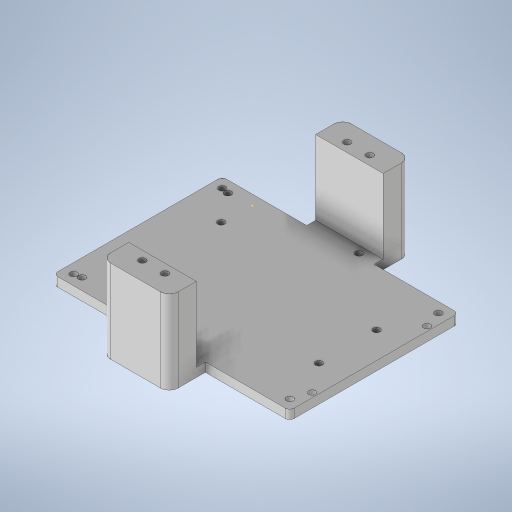
# Autodesk Inventor part: pablo opencr
Saved by Autodesk Inventor 2023 (Build 270158000, 158)
## iProperties
Created: 2022-09-07
Part Number: pablo opencr
Material: Genérico
Document SubType Name: Modeling
Designer: Lab. de Manufactura
Density: 1 g/cm^3
Appearance: Valor por defecto
Author: Lab. de Manufactura
Autodesk Inventor part; units mm, degrees
ref_plane "YZ Plane" through (0, 0, 0) normal (1, 0, 0) x (0, 1, 0)
ref_plane "XZ Plane" through (0, 0, 0) normal (0, 1, 0) x (-1, 0, 0)
ref_plane "XY Plane" through (0, 0, 0) normal (0, 0, 1) x (1, 0, 0)
sketch "Boceto1" plane through (0, 0, 0) normal (0, 1, 0) x (-1, 0, 0)
  line L0 (0, 0) -> (0, -87) construction
  line L1 (0, 0) -> (0, 83.8978) construction
  line L2 (0, 0) -> (-87, 0) construction
  line L3 (0, 0) -> (59, 0) construction
  line L4 (-74.5, -10) -> (-49.5, -10)
  line L5 (-49.5, -10) -> (-49.5, 10)
  line L6 (-49.5, 10) -> (-74.5, 10)
  line L7 (-74.5, 10) -> (-74.5, -10)
  line L8 (-74.5, -10) -> (-49.5, 10) construction
  line L9 (-49.5, -10) -> (-74.5, 10) construction
  line L10 (-18, 63.0769) -> (-64.0145, 27.7688)
  line L11 (9, 69.9829) -> (55.0145, 34.6747)
  line L12 (9, 69.9829) -> (20.2282, 84.6157)
  line L13 (-18, 63.0769) -> (-31.752, 80.9988)
  line L14 (-64.0145, 27.7688) -> (-75.6609, 42.9467)
  line L15 (-18, -63.0769) -> (-64.0145, -27.7688)
  line L16 (9, -69.9829) -> (55.0145, -34.6747)
  line L17 (9, -69.9829) -> (20.2282, -84.6157)
  line L18 (-18, -63.0769) -> (-31.752, -80.9988)
  line L19 (-64.0145, -27.7688) -> (-75.6609, -42.9467)
  arc A0 (-75.6609, 42.9467) -> (-75.6609, -42.9467) centre (0, 0) ccw
  arc A1 (20.2282, 84.6157) -> (-31.752, 80.9988) centre (0, 0) ccw
  arc A2 (-31.752, -80.9988) -> (20.2282, -84.6157) centre (0, 0) ccw
  line L20 (59, 37.9189) -> (59, -37.9189)
  line L21 (58.0583, 38.6415) -> (59, 37.9189)
  line L22 (55.0145, 34.6747) -> (58.0583, 38.6415)
  line L23 (58.0583, -38.6415) -> (59, -37.9189)
  line L24 (55.0145, -34.6747) -> (58.0583, -38.6415)
  circle A3 centre (-18.868, 51.0667) radius 1.5
  circle A4 centre (-52.1888, 25.4987) radius 1.5
  line L25 (-41.0072, 45.4229) -> (-35.5284, 38.2827) construction
  line L26 (-18.868, 51.0667) -> (-52.1888, 25.4987) construction
  line L27 (32.0072, 52.3288) -> (22.9685, 40.5493) construction
  circle A5 centre (9.868, 57.9726) radius 1.5
  circle A6 centre (43.1888, 32.4046) radius 1.5
  circle A7 centre (-18.868, -51.0667) radius 1.5
  circle A8 centre (-52.1888, -25.4987) radius 1.5
  circle A9 centre (9.868, -57.9726) radius 1.5
  circle A10 centre (43.1888, -32.4046) radius 1.5
  line L28 (43.1888, 32.4046) -> (9.868, 57.9726) construction
  point P0 (-62, 0)
  point P1 (-74.5, 0)
  point P2 (26.5284, 45.1886)
  dimension "d1" = 25
  dimension "d2" = 20
  dimension "d9" = 52.5
  dimension "d10" = 52.5
  dimension "d11" = 61
  dimension "d12" = 61
  dimension "d13" = 58
  dimension "d17" = 90
  dimension "d18" = 9
  dimension "d19" = 18
  dimension "d20" = 58
  dimension "d21" = 90
  dimension "d22" = 90
  dimension "d23" = 87
  dimension "d24" = 87
  dimension "d26" = 59
  dimension "d27" = 5
  dimension "d28" = 5
  dimension "d29" = 3
  dimension "d30" = 3
  dimension "d31" = 42
  dimension "d32" = 9
  dimension "d37" = 90
  dimension "d38" = 3
  dimension "d39" = 3
  dimension "d40" = 42
  dimension "d41" = 9
  dimension "d54" = 62
  constraints: 58 end point, 11 centre point, 11 symmetric about line, 9 parallel, 8 point on circle, 7 midpoint, 3 horizontal, 3 vertical, 2 perpendicular, 2 point on line, 1 coincident, 4 other
  measures "d1" distance of L5.end L6.end
  measures "d2" distance of L4.end L5.end
  measures "d9" angle of L1 L11
  measures "d10" angle of L1 L10
  measures "d11" distance from line of point (0, 0) L11
  measures "d12" distance from line of point (0, 0) L10
  measures "d13" distance of L11.start L11.end
  measures "d17" angle of L11 L12
  measures "d18" distance from line of L1 L11.start
  measures "d19" distance from line of L1 L10.start
  measures "d20" distance of L10.start L10.end
  measures "d21" angle of L10 L13
  measures "d22" angle of L10 L14
  measures "d23" radius of A0
  measures "d24" radius of A1
  measures "d26" distance between parallel lines of L0 L20
  measures "d27" distance between parallel lines of L11 L21
  measures "d28" distance between parallel lines of L23 L16
  measures "d29" diameter of A3
  measures "d30" diameter of A4
  measures "d31" distance of L26.end L26.start
  measures "d32" distance from line of L10 L26.start
  measures "d37" angle of L11 L27
  measures "d38" diameter of A5
  measures "d39" diameter of A6
  measures "d40" distance of L28.end L28.start
  measures "d41" distance from line of L11 L28.end
  measures "d54" distance of point (0, 0) point (-62, 0)
extrude "Extrusión1" add sketch "Boceto1" along normal blind 3
sketch "Boceto2" plane through (0, 3, 0) normal (0, 1, 0) x (1, 0, 0)
  line L0 (-55.0145, -34.6747) -> (-9, -69.9829) projected
  line L1 (-32.0072, -52.3288) -> (-0.1642, -10.8301) construction
  circle A0 centre (-33.4486, -19.711) radius 1.55
  circle A1 centre (-0.1278, -45.2789) radius 1.55
  line L2 (-33.4486, -19.711) -> (-0.1278, -45.2789) construction
  circle A2 centre (-43.1888, -32.4046) radius 1.5 construction
  line L3 (18, -63.0769) -> (64.0145, -27.7688) projected
  line L4 (41.0072, -45.4229) -> (14.3892, -10.7335) construction
  circle A3 centre (9.1278, -38.373) radius 1.55
  circle A4 centre (42.4486, -12.805) radius 1.55
  line L5 (42.4486, -12.805) -> (9.1278, -38.373) construction
  circle A5 centre (18.868, -51.0667) radius 1.5 construction
  line L6 (-59, 37.9189) -> (-59, -37.9189) construction
  line L7 (-59, 0) -> (115.874, 0) construction
  circle A6 centre (-33.4486, 19.711) radius 1.55
  circle A7 centre (-0.1278, 45.2789) radius 1.55
  circle A8 centre (9.1278, 38.373) radius 1.55
  circle A9 centre (42.4486, 12.805) radius 1.55
  point P0 (0, 0)
  dimension "d44" = 3.1
  dimension "d45" = 3.1
  dimension "d46" = 21
  dimension "d47" = 42
  dimension "d48" = 16
  dimension "d51" = 16
  dimension "d52" = 21
  dimension "d53" = 42
  constraints: 10 end point, 8 centre point, 4 symmetric about line, 3 midpoint, 2 equal radius, 2 parallel, 2 perpendicular, 1 horizontal, 4 other
  measures "d44" diameter of A0
  measures "d45" diameter of A1
  measures "d46" distance from line of L1 L2.start
  measures "d47" distance of L2.start L2.end
  measures "d48" distance of A2.centre L2.start
  measures "d51" distance from line of L5 A5.centre
  measures "d52" distance from line of L4 L5.end
  measures "d53" distance of L5.start L5.end
extrude "Extrusión2" cut sketch "Boceto2" against normal blind 10
sketch "Boceto3" plane through (0, 3, 0) normal (0, 1, 0) x (1, 0, 0)
  circle A0 centre (0, 0) radius 90 construction
  dimension "d55" = 180
  constraints: 1 centre point, 1 coincident
  measures "d55" diameter of A0
sketch "Boceto5" plane through (0, 3, 0) normal (0, 1, 0) x (1, 0, 0)
  arc A0 (75.6609, -42.9467) -> (75.6609, 42.9467) centre (0, 0) ccw construction
  line L0 (87, 0) -> (-107.1861, 0) construction
  line L1 (-55.0145, -34.6747) -> (-9, -69.9829) projected
  line L2 (-9, -69.9829) -> (5.2804, -80.9406)
  line L3 (5.2804, -80.9406) -> (0.6326, -86.9977)
  arc A1 (-20.2282, -84.6157) -> (31.752, -80.9988) centre (0, 0) ccw projected
  line L4 (31.752, -80.9988) -> (18, -63.0769) projected
  line L5 (18, -63.0769) -> (4.513, -73.4259)
  line L6 (4.513, -73.4259) -> (9.3831, -79.7727)
  line L7 (9.3831, -79.7727) -> (22.8701, -69.4238)
  line L8 (-55.0145, -34.6747) -> (-59, -31.6165)
  line L9 (-59, 37.9189) -> (-59, -37.9189) projected
  circle A2 centre (42.4486, 12.805) radius 1.55 projected
  circle A3 centre (-33.4486, -19.711) radius 1.55 projected
  circle A4 centre (-33.4486, 19.711) radius 1.55 projected
  circle A5 centre (42.4486, -12.805) radius 1.55 projected
  circle A6 centre (9.1278, 38.373) radius 1.55 projected
  circle A7 centre (-0.1278, -45.2789) radius 1.55 projected
  circle A8 centre (-0.1278, 45.2789) radius 1.55 projected
  circle A9 centre (9.1278, -38.373) radius 1.55 projected
  arc A10 (-20.2282, -84.6157) -> (31.752, -80.9988) centre (0, 0) ccw projected
  line L10 (31.752, -80.9988) -> (18, -63.0769) projected
  line L11 (18, -63.0769) -> (64.0145, -27.7688) projected
  line L12 (64.0145, -27.7688) -> (75.6609, -42.9467) projected
  arc A11 (75.6609, -42.9467) -> (75.6609, 42.9467) centre (0, 0) ccw projected
  line L13 (75.6609, 42.9467) -> (64.0145, 27.7688) projected
  line L14 (64.0145, 27.7688) -> (18, 63.0769) projected
  line L15 (18, 63.0769) -> (31.752, 80.9988) projected
  arc A12 (31.752, 80.9988) -> (-20.2282, 84.6157) centre (0, 0) ccw projected
  line L16 (-20.2282, 84.6157) -> (-9, 69.9829) projected
  line L17 (-9, 69.9829) -> (-55.0145, 34.6747) projected
  line L18 (-55.0145, 34.6747) -> (-58.0583, 38.6415) projected
  line L19 (-58.0583, 38.6415) -> (-59, 37.9189) projected
  line L20 (-59, 37.9189) -> (-59, -37.9189) projected
  line L21 (-59, -37.9189) -> (-58.0583, -38.6415) projected
  line L22 (-58.0583, -38.6415) -> (-55.0145, -34.6747) projected
  line L23 (-55.0145, -34.6747) -> (-9, -69.9829) projected
  line L24 (-9, -69.9829) -> (-20.2282, -84.6157) projected
  circle A13 centre (-43.1888, 32.4046) radius 1.5 projected
  circle A14 centre (-9.868, 57.9726) radius 1.5 projected
  circle A15 centre (18.868, 51.0667) radius 1.5 projected
  circle A16 centre (52.1888, 25.4987) radius 1.5 projected
  circle A17 centre (-43.1888, -32.4046) radius 1.5 projected
  circle A18 centre (-9.868, -57.9726) radius 1.5 projected
  circle A19 centre (52.1888, -25.4987) radius 1.5 projected
  circle A20 centre (18.868, -51.0667) radius 1.5 projected
  line L25 (74.5, 10) -> (74.5, -10) projected
  line L26 (74.5, -10) -> (49.5, -10) projected
  line L27 (49.5, -10) -> (49.5, 10) projected
  line L28 (49.5, 10) -> (74.5, 10) projected
  line L29 (18, -63.0769) -> (64.0145, -27.7688) projected
  line L30 (64.0145, -27.7688) -> (78.2949, -16.8111)
  line L31 (78.2949, -16.8111) -> (83.6749, -23.8225)
  point P0 (-9, -69.9829)
  point P1 (-20.2282, -84.6157)
  dimension "d66" = 18
  dimension "d67" = 17
  dimension "d68" = 8
  dimension "d69" = 18
  constraints: 18 end point, 5 perpendicular, 3 collinear, 3 point on circle, 2 point on line, 1 horizontal
  measures "d66" distance of L1.end L2.end
  measures "d67" distance of L4.end L5.end
  measures "d68" distance of L5.end L6.end
  measures "d69" distance of L11.end L30.end
extrude "Extrusión3" cut sketch "Boceto5" against normal blind 10 contours L22 L21 L9 L8 | L2 L3 A1 L24 | L7 L6 L5 L4 | L30 L31 A11 L12
mirror "Simetría1" about plane through (0, 0, 0) normal (0, 0, 1) of "Extrusión3"
sketch "Boceto6" plane through (0, 3, 0) normal (0, 1, 0) x (1, 0, 0)
  line L0 (-59, 31.6165) -> (-59, -31.6165) projected
  line L1 (-59, 0) -> (-50.8, 0)
  line L2 (-50.8, 0) -> (-50.8, 35.5)
  line L3 (-48.8, 37.5) -> (52.2, 37.5)
  line L4 (54.2, 35.5) -> (54.2, -35.5)
  line L5 (-50.8, 0) -> (-50.8, -35.5)
  line L6 (-48.8, -37.5) -> (52.2, -37.5)
  arc A0 (-50.8, -35.5) -> (-48.8, -37.5) centre (-48.8, -35.5) ccw
  arc A1 (-48.8, 37.5) -> (-50.8, 35.5) centre (-48.8, 35.5) ccw
  arc A2 (54.2, 35.5) -> (52.2, 37.5) centre (52.2, 35.5) ccw
  arc A3 (52.2, -37.5) -> (54.2, -35.5) centre (52.2, -35.5) ccw
  point P0 (0, 0)
  point P1 (-50.8, 37.5)
  point P2 (54.2, 37.5)
  point P3 (54.2, -37.5)
  point P4 (-50.8, -37.5)
  dimension "d72" = 8.2
  dimension "d73" = 37.5
  dimension "d74" = 105
  dimension "d75" = 75
  dimension "d76" = 37.5
  dimension "d77" = 105
  dimension "d78" = 2
  constraints: 12 end point, 8 point on circle, 8 point on line, 8 tangent, 4 centre point, 3 equal radius, 2 horizontal, 2 vertical, 1 midpoint, 1 perpendicular
  measures "d72" distance of L1.start L1.end
  measures "d73" distance of L1.end point (-50.8, 37.5)
  measures "d74" distance of point (-50.8, 37.5) point (54.2, 37.5)
  measures "d75" distance of point (54.2, 37.5) point (54.2, -37.5)
  measures "d76" distance of L1.end point (-50.8, -37.5)
  measures "d77" distance of point (-50.8, -37.5) point (54.2, -37.5)
  measures "d78" radius of A0
extrude "Extrusión4" add sketch "Boceto6" along normal blind 4
sketch "Boceto7" plane through (0, 0, 0) normal (0, -1, 0) x (1, 0, 0)
  circle A0 centre (-33.4486, -19.711) radius 1.55 projected
  circle A1 centre (-33.4486, -19.711) radius 1.55
  circle A2 centre (-43.1888, -32.4046) radius 1.5 projected
  circle A3 centre (-43.1888, -32.4046) radius 1.5
  circle A4 centre (-33.4486, 19.711) radius 1.55 projected
  circle A5 centre (-33.4486, 19.711) radius 1.55
  circle A6 centre (-43.1888, 32.4046) radius 1.5 projected
  circle A7 centre (-43.1888, 32.4046) radius 1.5
  circle A8 centre (9.1278, 38.373) radius 1.55 projected
  circle A9 centre (9.1278, 38.373) radius 1.55
  circle A10 centre (9.1278, -38.373) radius 1.55 projected
  circle A11 centre (9.1278, -38.373) radius 1.55
  circle A12 centre (42.4486, -12.805) radius 1.55 projected
  circle A13 centre (42.4486, -12.805) radius 1.55
  circle A14 centre (42.4486, 12.805) radius 1.55 projected
  circle A15 centre (42.4486, 12.805) radius 1.55
  circle A16 centre (52.1888, -25.4987) radius 1.5 projected
  circle A17 centre (52.1888, -25.4987) radius 1.5
  circle A18 centre (52.1888, 25.5678) radius 1.5016
  point P0 (0, 0)
  dimension "d81" = 3.0032
  dimension "d82" = 3
  dimension "d83" = 3.1
  dimension "d84" = 3.1
  dimension "d85" = 3.1
  dimension "d86" = 3.1
  dimension "d87" = 3.1
  dimension "d88" = 3.1
  dimension "d89" = 3
  dimension "d90" = 3
  dimension "d91" = 51.0664
  dimension "d92" = 16.0549
  constraints: 10 centre point, 9 coincident
  measures "d81" diameter of A18
  measures "d82" diameter of A17
  measures "d83" diameter of A15
  measures "d84" diameter of A13
  measures "d85" diameter of A9
  measures "d86" diameter of A11
  measures "d87" diameter of A5
  measures "d88" diameter of A1
  measures "d89" diameter of A7
  measures "d90" diameter of A3
  measures "d91" distance of A16.centre A18.centre
  measures "d92" distance of A14.centre A18.centre
hole "Agujero1" at (-43.1888, 0, -32.4046) at (-33.4486, 0, -19.711) at (-33.4486, 0, 19.711) at (-43.1888, 0, 32.4046) at (9.1278, 0, -38.373) at (42.4486, 0, -12.805) at (42.4486, 0, 12.805) at (52.1888, 0, 25.5678) at (9.1278, 0, 38.373) direction (0, 1, 0) diameter 3 end through all
sketch "Boceto8" plane through (0, 0, 0) normal (0, -1, 0) x (1, 0, 0)
  circle A0 centre (52.1888, -25.4987) radius 1.5 projected
  circle A1 centre (52.1888, -25.4987) radius 1.5
  point P0 (0, 0)
  constraints: 1 centre point, 1 coincident
hole "Agujero2" at (52.1888, 0, -25.4987) direction (0, 1, 0) diameter 3 end through all
sketch "Boceto9" plane through (0, 7, 0) normal (0, 1, 0) x (1, 0, 0)
  circle A0 centre (-46.3, -33.001) radius 2
  line L0 (0, 0) -> (-50.8, 0)
  line L1 (-50.8, 35.5) -> (-50.8, -35.5) projected
  line L2 (0, 0) -> (54.2, 0)
  line L3 (54.2, -10) -> (54.2, 10) projected
  line L4 (0, 0) -> (0, -37.5107)
  line L5 (-50.8, 0) -> (-50.8, -35.5)
  line L6 (-48.8, -37.5) -> (7.908, -37.5) projected
  circle A1 centre (-46.3, 33.001) radius 2
  line L7 (54.2, -10) -> (54.2, -35.2997) projected
  circle A2 centre (49.7, -33) radius 2
  circle A3 centre (49.7, 33) radius 2
  dimension "d109" = 4
  dimension "d114" = 4
  dimension "d118" = 4.5
  dimension "d119" = 70.5
  dimension "d120" = 0.0107
  dimension "d121" = 100.5
  dimension "d122" = 70.501
  constraints: 8 end point, 4 centre point, 2 midpoint, 2 symmetric about line, 2 vertical, 2 other
  measures "d109" diameter of A0
  measures "d114" diameter of A2
  measures "d118" distance from line of A3.centre L3
  measures "d119" distance from line of A3.centre L6
  measures "d120" distance from line of L4.end L6
  measures "d121" distance from line of A1.centre L3
  measures "d122" distance from line of A1.centre L6
hole "Agujero3" at (-46.3, 7, -33.001) at (-46.3, 7, 33.001) at (49.7, 7, -33) at (49.7, 7, 33) direction (0, -1, 0) diameter 3 end through all
sketch "Boceto10" plane through (-59, 0, -31.6165) normal (-1, 0, 0) x (0, 0, 1)
  line L0 (-49.3823, 0) -> (-55.3812, 0) projected
  line L1 (118.6142, 3) -> (118.6142, 0) projected
  line L2 (-55.3812, 0) -> (118.6142, 0)
  line L3 (118.6142, 0) -> (118.6142, 3)
  line L4 (118.6142, 3) -> (-55.3812, 3)
  line L5 (-55.3812, 3) -> (-55.3812, 0)
  point P0 (31.6165, 0)
  point P1 (-49.3823, 0)
  constraints: 8 end point, 2 parallel, 1 horizontal, 1 perpendicular
extrude "Extrusión5" cut sketch "Boceto10" against normal blind 1000
sketch "Boceto11" plane through (-48.8, 3, 37.5) normal (0, 0, 1) x (1, 0, 0)
  line L0 (-2, 0) -> (0, 0) projected
  line L1 (-2, 0) -> (50.5, 0)
  line L2 (56.708, 0) -> (0, 0) construction
  line L3 (50.5, 0) -> (65.5, 0)
  line L4 (50.5, 0) -> (35.5, 0) construction
  line L5 (103, 4) -> (101, 4) projected
  line L6 (103, 4) -> (-2, 4) construction
  line L7 (65.5, 0) -> (65.5, 4)
  line L8 (35.5, 0) -> (35.5, 4)
  line L9 (56.708, 4) -> (0, 4) projected
  line L10 (35.5, 0) -> (50.5, 0)
  line L11 (35.5, 4) -> (65.5, 4)
  line L12 (101, 4) -> (59.1476, 4) projected
  point P0 (48.8, -3)
  point P1 (35.5, 0)
  dimension "d132" = 52.5
  dimension "d133" = 15
  dimension "d134" = 15
  constraints: 16 end point, 4 point on line, 3 horizontal, 2 perpendicular, 1 collinear
  measures "d132" distance of L0.start L1.end
  measures "d133" distance of L1.end L3.end
  measures "d134" distance of L1.end L4.end
extrude "Extrusión6" add sketch "Boceto11" along normal blind 16
sketch "Boceto12" plane through (0, 7, 0) normal (0, 1, 0) x (1, 0, 0)
  line L0 (-50.8, -35.5) -> (-50.8, 35.5) projected
  line L1 (-50.8, 0) -> (54.2, 0)
  line L2 (54.2, -35.5) -> (54.2, 35.5) projected
  line L3 (-13.3, -37.5) -> (-13.3, -53.5) projected
  line L4 (-13.3, -37.5) -> (-13.3, -53.5)
  line L5 (-13.3, -53.5) -> (16.7, -53.5) projected
  line L6 (-13.3, -53.5) -> (16.7, -53.5)
  line L7 (16.7, -53.5) -> (16.7, -37.5)
  line L8 (16.7, -37.5) -> (-13.3, -37.5)
  line L9 (-13.3, 37.5) -> (-13.3, 53.5)
  line L10 (-13.3, 53.5) -> (16.7, 53.5)
  line L11 (16.7, 53.5) -> (16.7, 37.5)
  line L12 (16.7, 37.5) -> (-13.3, 37.5)
  point P0 (0, 0)
  constraints: 18 end point, 4 symmetric about line, 3 perpendicular, 2 midpoint, 1 vertical
extrude "Extrusión7" add sketch "Boceto12" against normal blind 4 contours L9 L10 L11 L12
sketch "Boceto13" plane through (0, 7, 0) normal (0, 1, 0) x (1, 0, 0)
  arc A0 (10.3476, -37.5) -> (7.908, -37.5) centre (9.1278, -38.373) ccw projected
  circle A1 centre (9.1278, -38.373) radius 1.5
  line L0 (0, 0) -> (5.9834, 0)
  circle A2 centre (9.1278, 38.373) radius 1.5
  dimension "d139" = 3
  constraints: 2 centre point, 2 end point, 1 coincident, 1 horizontal, 1 symmetric about line, 1 other
  measures "d139" diameter of A1
extrude "Extrusión8" cut sketch "Boceto13" against normal blind 4
sketch "Boceto14" plane through (0, 7, 0) normal (0, 1, 0) x (1, 0, 0)
  line L0 (-13.3, -37.5) -> (-13.3, -53.5) projected
  line L1 (-13.3, -53.5) -> (-13.3, -41.5)
  line L2 (-13.3, -41.5) -> (16.7, -41.5)
  line L3 (16.7, -37.5) -> (16.7, -53.5) projected
  line L4 (-13.3, -53.5) -> (16.7, -53.5)
  line L5 (16.7, -53.5) -> (16.7, -41.5)
  line L6 (0, 0) -> (-15.8306, 0)
  line L7 (16.7, -41.5) -> (16.7, -53.5)
  line L8 (-13.3, 37.5) -> (-13.3, 53.5)
  line L9 (-13.3, 41.5) -> (16.7, 41.5)
  line L10 (16.7, 37.5) -> (16.7, 53.5)
  line L11 (-13.3, 53.5) -> (16.7, 53.5)
  dimension "d142" = 12
  constraints: 20 end point, 6 symmetric about line, 4 point on line, 3 perpendicular, 1 horizontal, 1 vertical
  measures "d142" distance of L0.end L1.end
extrude "Extrusión9" add sketch "Boceto14" along normal blind 33
sketch "Boceto15" plane through (0, 40, 0) normal (0, 1, 0) x (1, 0, 0)
  point P0 (0, 0)
sketch "Boceto16" plane through (0, 40, 0) normal (0, 1, 0) x (1, 0, 0)
  point P0 (0, 0)
fillet "Empalme1" radius 4 4 edges at (16.7, 21.5, -53.5) (-13.3, 21.5, -53.5) (16.7, 21.5, 53.5) (-13.3, 21.5, 53.5)
sketch "Boceto17" plane through (12.7, 40, -53.5) normal (0, 0, -1) x (-1, 0, 0)
  line L0 (0, 0) -> (22, 0) projected
  line L1 (11, 0) -> (11, -37)
  line L2 (22, -37) -> (0, -37) projected
  line L3 (11, -18.5) -> (22, -18.5)
  line L4 (22, 0) -> (22, -37) projected
  line L5 (11, 0) -> (11, -18.5)
  circle A0 centre (11, -9.25) radius 2
  point P0 (12.7, -40)
  dimension "d146" = 4
  constraints: 6 end point, 5 midpoint, 1 centre point, 1 vertical
  measures "d146" diameter of A0
hole "Agujero4" at (1.7, 30.75, -53.5) direction (0, 0, 1) diameter 3 depth 4 tip angle 118
sketch "Boceto18" plane through (0, 40, 0) normal (0, 1, 0) x (1, 0, 0)
  line L0 (-13.3, 41.5) -> (16.7, 41.5) projected
  line L1 (-13.3, 41.5) -> (16.7, 41.5)
  line L2 (16.7, 41.5) -> (16.7, 49.5)
  line L3 (-13.3, 49.5) -> (-13.3, 41.5) projected
  line L4 (16.7, 49.5) -> (-13.3, 49.5)
  line L5 (16.7, 45.5) -> (-13.3, 45.5)
  line L6 (-13.3, 45.5) -> (-3.3, 45.5)
  circle A0 centre (-3.3, 45.5) radius 1.5
  line L7 (16.7, 45.5) -> (6.7, 45.5)
  circle A1 centre (6.7, 45.5) radius 1.5
  line L8 (53.6389, 0) -> (-50.8, 0)
  line L9 (-50.8, -35.5) -> (-50.8, 35.5) projected
  circle A2 centre (-3.3, -45.5) radius 1.5
  circle A3 centre (6.7, -45.5) radius 1.5
  point P0 (0, 0)
  dimension "d154" = 10
  dimension "d155" = 3
  dimension "d156" = 10
  dimension "d157" = 3
  constraints: 14 end point, 4 centre point, 3 midpoint, 2 coincident, 2 perpendicular, 2 point on line, 2 symmetric about line, 1 horizontal, 2 other
  measures "d154" distance of L5.end L6.end
  measures "d155" diameter of A0
  measures "d156" distance of L5.start L7.end
  measures "d157" diameter of A1
extrude "Extrusión10" cut sketch "Boceto18" against normal blind 13 contours A0 L5 | L5 A0 | A1 L5 | L5 A1 | A2 | A3
ref_plane "Plano de trabajo1" through (0, 0, 0) normal (0, 0, 1) x (1, 0, 0)
